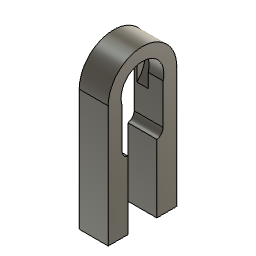
Wedge Stand (Autodesk Fusion 360 design; units mm, degrees)
Autodesk Fusion 360 part; units mm, degrees
note: some values were not read from the file. Chosen so that the rebuilt part matches the saved one: which bodies a step acts on; which face or edge a step refers to; which pieces of a blend or face edit are solid. Set by a fixed rule: which sketch regions a step uses.
sketch "Sketch1" plane through (0, 0, 0) normal (0, 1, 0) x (1, 0, 0)
sketch "Sketch2" plane through (0, 0, 0) normal (1, 0, 0) x (0, 1, 0)
  circle A0 centre (0, 0) radius 19.8222
  circle A1 centre (0, 0) radius 23.6949
  line L0 (14.2611, -13.9074) -> (14.2611, -24.9053)
  line L1 (14.2611, -24.9053) -> (-14.1247, -24.9053)
  line L2 (-14.1247, -24.9053) -> (-14.1247, -13.9074)
  line L3 (0, 0) -> (23.6949, 0)
  line L4 (0, 0) -> (-23.6949, 0)
  line L5 (-23.6949, 0) -> (23.6951, 0)
  line L6 (23.6951, 0) -> (23.6951, -70.1053)
  line L7 (23.6951, -70.1053) -> (-23.6949, -70.1053)
  line L8 (-23.6949, -70.1053) -> (-23.6949, 0)
  line L9 (-10.0299, -70.1053) -> (9.9161, -70.1053)
  line L10 (9.9161, -70.1053) -> (9.9161, -40.1053)
  line L11 (9.9161, -40.1053) -> (-10.0299, -40.1053)
  line L12 (-10.0299, -40.1053) -> (-10.0299, -70.1053)
  dimension "d1" = 47.39
  dimension "d2" = 19.946
  dimension "d3" = 30
  constraint coincident A0.centre A1.centre
  constraint concentric A0 A1
  constraint vertical L0
  constraint horizontal L1
  constraint vertical L2
  constraint coincident A0 L2.end
  constraint coincident A1 L3.end
  constraint horizontal L3
  constraint coincident A1 L4.end
  constraint parallel L3 L4
  constraint horizontal L5
  constraint vertical L6
  constraint horizontal L7
  constraint vertical L8
  constraint horizontal L9
  constraint vertical L10
  constraint horizontal L11
  constraint vertical L12
  constraint coincident L7 L9.start
  measures "d1" distance of L4.end L5.end
  measures "d2" distance of L9.start L9.end
  measures "d3" distance of L9.start L11.end
extrude "Extrude1" add sketch "Sketch2" along normal blind 20 contours A0 A1 L2 L4 L5 | A0 A1 L2 L3 L5 | A0 A1 L3 L4 L5 | A1 L0 L1 L2 L6 L7 L8 L10 L11 L12 | A1 L0 L1 L2 makes body 1
split "Split1" by curves path "Sketch2" along A1 bodies 1 makes body 2 at (0, -0.6282, -34.6131)
split "Split2" by curves path "Sketch2" along L0 L1 L2 bodies 2 makes body 3 at (0, 3.3508, -29.9719)
split "Split3" by curves path "Sketch2" along L0 L1 L2 bodies 1 makes body 4 at (13.3333, 13.5787, -14.4409) makes body 5 at (13.3333, -17.966, -15.4489) makes body 6 at (13.3333, 15.0804, -18.2764)
combine "Combine1" operation add target body 4 tool bodies 2
combine "Combine2" operation add target body 6 tool bodies 1
combine "Combine3" operation add target body 6 tool bodies 5
combine "Combine4" operation add target body 6 tool bodies 3
extrude "Extrude2" cut 1 faces at (6.6667, 3.2674, -40.1053) along direction (0, 0, 1) blind 25 on bodies 6 bodies 4 6 makes body 7 at (6.6667, -14.1247, -21.2393)
extrude "Extrude3" cut 2 faces at (0, 11.3644, -22.3247) (0, -11.3948, -22.3026) along direction (1, 0, 0) blind 25 on bodies 4 7 bodies 4 7
extrude "Extrude4" cut 2 faces at (13.3333, -11.3948, -24.9053) (6.6667, 12.8127, -24.9053) along direction (0, 0, -1) blind 12 on bodies 6 bodies 6
extrude "Extrude5" cut 1 faces at (20, 15.9574, -59.0386) along direction (-1, 0, 0) blind 10 on bodies 6 bodies 6
extrude "Extrude6" cut 2 faces at (3.3333, -14.5849, -70.1053) (3.3333, 19.1021, -70.1053) along direction (0, 0, 1) blind 11.2 on bodies 6 bodies 6
sketch "Sketch3" plane through (10, 0, 0) normal (1, 0, 0) x (0, 1, 0)
  line L0 (-23.6949, -58.9053) -> (-10.0299, -58.9053)
  line L1 (-10.0299, -58.9053) -> (-10.0299, -36.9053)
  line L2 (-10.0299, -36.9053) -> (-14.1247, -36.9053)
  line L3 (-14.1247, -36.9053) -> (-14.1247, -13.9074)
  arc A0 (14.2611, -13.7674) -> (-14.1247, -13.9074) centre (0, 0) ccw
  line L4 (14.2611, -13.7674) -> (14.2611, -36.9053)
  line L5 (14.2611, -36.9053) -> (9.9161, -36.9053)
  line L6 (9.9161, -36.9053) -> (9.9161, -58.9053)
  line L7 (9.9161, -58.9053) -> (23.6951, -58.9053)
  line L8 (23.6951, -58.9053) -> (23.6951, 0)
  line L9 (23.6951, 0) -> (23.6949, 0)
  arc A1 (23.6949, 0) -> (-23.6949, 0) centre (0, 0) ccw
  line L10 (-23.6949, 0) -> (-23.6949, -58.9053)
sketch "Sketch4" plane through (0, 0, 0) normal (0, 0.92388, -0.382683) x (-1, 0, 0)
  line L0 (0, 15.875) -> (0, 18.875)
  line L1 (0, 18.875) -> (-6.35, 18.875)
  line L2 (-6.35, 18.875) -> (-6.35, 15.875)
  line L3 (-6.35, 15.875) -> (0, 15.875)
  line L4 (-8.7684, 25.1445) -> (-8.7684, -15)
  constraint vertical L4
split "Split4" by curves path "Sketch4" along L4 bodies 6 makes body 8 at (10, 15.9574, -51.5719)
move_face "OffsetFaces1" offset 1 1 faces at (9.5895, -16.7752, -10.56) on bodies 8
combine "Combine5" operation add target body 6 tool bodies 8
extrude "Extrude7" add 2 faces at (6.6667, 14.5091, -58.9053) (3.3333, -14.5849, -58.9053) along direction (0, 0, -1) blind 25 on bodies 6 bodies 6 4 7
extrude "Extrude8" add 1 faces at (0, 14.5091, -59.9053) along direction (-1, 0, 0) blind 10 on bodies 6 bodies 6
extrude "Extrude9" add 1 faces at (8.7684, 2.7038, 18.9293) along direction (-1, 0, 0) blind 6 on bodies 6 bodies 6
sketch "Sketch5" plane through (0, 0, 0) normal (0, 0.707107, -0.707107) x (-1, 0, 0)
  line L0 (8, 15.875) -> (8, 18.875)
  line L1 (8, 18.875) -> (1.65, 18.875)
  line L2 (1.65, 18.875) -> (1.65, 15.875)
  line L3 (1.65, 15.875) -> (8, 15.875)
  line L4 (8, 34) -> (8, 5.461)
  constraint vertical L4
split "Split5" by curves path "Sketch5" along L4 bodies 6 makes body 9 at (10, -15.9498, -69.2386)
move_face "OffsetFaces2" offset 5 1 faces at (-9.3333, 1.3495, 19.7762) on bodies 6
combine "Combine6" operation add target body 6 tool bodies 9
fillet "Fillet1" radius 5 2 edges at (0, 14.2611, -36.9053) (0, -14.1247, -36.9053) on bodies 6
move_face "OffsetFaces3" offset 4 1 faces at (5.1789, -18.758, -1.5532) on bodies 6
extrude "Extrude10" add 1 faces at (2.7684, 15.3838, -8.4622) along direction (-1, 0, 0) blind 3 on bodies 6 bodies 6
named bodies: "Wedge Stand"
